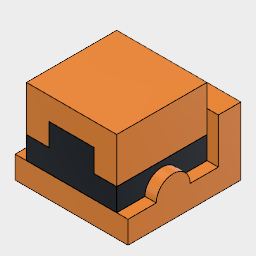
Tier 2 Practice Ex2_ CSA011070∩╗┐ (Autodesk Fusion 360 design; units mm, degrees)
Autodesk Fusion 360 part; units mm, degrees
note: some values were not read from the file. Set by a fixed rule: which sketch regions a step uses.
sketch "Sketch1" plane through (0, 0, 0) normal (0, 0, 1) x (1, 0, 0) in component "Component"
  line L0 (0, 0) -> (25.4, 0)
  line L1 (25.4, 0) -> (25.4, -25.4)
  line L2 (25.4, -25.4) -> (50.8, -25.4)
  line L3 (50.8, -25.4) -> (50.8, 25.4)
  line L4 (50.8, 25.4) -> (0, 25.4)
  line L5 (0, 25.4) -> (0, 0)
  line L6 (-50.8, 25.4) -> (0, 25.4)
  line L7 (-50.8, -25.4) -> (-50.8, 25.4)
  line L8 (-25.4, -25.4) -> (-50.8, -25.4)
  line L9 (-25.4, 0) -> (-25.4, -25.4)
  line L10 (0, 0) -> (-25.4, 0)
  dimension "d1" = 25.4
  dimension "d2" = 25.4
  dimension "d3" = 25.4
  dimension "d4" = 50.8
  measures "d1" distance of L0.start L0.end
  measures "d2" distance of L0.end L1.end
  measures "d3" distance of L1.end L2.end
  measures "d4" distance of L2.end L3.end
extrude "Extrude1" add sketch "Sketch1" along normal mid plane 101.6 makes body 1 in component "Component"
sketch "Sketch1 (2)" plane through (0, 0, 0) normal (0, 0, 1) x (1, 0, 0) in component "Component'"
  line L0 (-25.4, -25.4) -> (-25.4, 0)
  line L1 (-25.4, 0) -> (25.4, 0)
  line L2 (25.4, 0) -> (25.4, -25.4)
  line L3 (-50.8, -25.4) -> (-25.4, -25.4)
  line L4 (25.4, -25.4) -> (50.8, -25.4)
  line L5 (-50.8, -25.4) -> (-50.8, -50.8)
  line L6 (-50.8, -50.8) -> (50.8, -50.8)
  line L7 (50.8, -50.8) -> (50.8, -25.4)
  dimension "d7" = 25.4
  measures "d7" distance of L3.start L5.end
extrude "Extrude1'" add sketch "Sketch1 (2)" along normal mid plane 101.6 separate body makes body 2 in component "Component'"
sketch "Sketch2" plane through (0, 0, 0) normal (1, 0, 0) x (0, 0, -1) in component "Component'"
  circle A0 centre (0, -50.8) radius 19.05
  line L0 (50.8, -50.8) -> (-50.8, -50.8)
  dimension "d10" = 38.1
  measures "d10" diameter of A0
extrude "Extrude2" cut sketch "Sketch2" along normal mid plane 142.24 bodies 2 in component "Component'"
sketch "Sketch1 (3)" plane through (0, 0, 0) normal (1, 0, 0) x (0, 0, -1) in component "Component''"
  arc A0 (-19.05, -50.8) -> (19.05, -50.8) centre (0, -50.8) cw
  line L0 (19.05, -50.8) -> (50.8, -50.8)
  line L1 (-50.8, -50.8) -> (-19.05, -50.8)
  line L2 (50.8, -50.8) -> (50.8, 0)
  line L3 (50.8, 0) -> (76.2, 0)
  line L4 (76.2, 0) -> (76.2, -76.2)
  line L5 (76.2, -76.2) -> (-50.8, -76.2)
  line L6 (-50.8, -76.2) -> (-50.8, -50.8)
  point P0 (50.8, 0)
  dimension "d13" = 25.4
  dimension "d14" = 25.4
  measures "d13" distance of L5.end L1.start
  measures "d14" distance of P0 L3.end
extrude "Extrude1''" add sketch "Sketch1 (3)" along normal mid plane 127 separate body makes body 3 in component "Component''"
component "Component" placed x (1, 0, 0) y (0, 1, 0) z (0, 0, 1) at (0, 0, 0)
component "Component'" placed x (1, 0, 0) y (0, 1, 0) z (0, 0, 1) at (0, 0, 0)
component "Component''" placed x (1, 0, 0) y (0, 1, 0) z (0, 0, 1) at (0, 0, 0)
